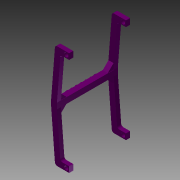
# Autodesk Inventor part: spac
Saved by Autodesk Inventor 2015 (Build 190159000, 159)
## iProperties
Created: 2015-01-15
Part Number: spac
Material: Generic
Document SubType Name: Modeling
Designer: Rafi Kurnia Putra
Density: 1 g/cm^3
Appearance: Smooth - Purple
Author: Rafi Kurnia Putra
Autodesk Inventor part; units mm, degrees
ref_plane "XZ Plane" through (0, 0, 0) normal (0, 1, 0) x (-1, 0, 0)
sketch "Sketch1" plane through (0, 0, 0) normal (0, 1, 0) x (-1, 0, 0)
  circle A0 centre (22.875, -42.175) radius 1.75
  line L0 (20.375, -39.675) -> (20.375, -44.675)
  line L1 (20.375, -44.675) -> (25.375, -44.675)
  line L2 (25.375, -44.675) -> (22.875, -44.675)
  line L3 (30.886, 0) -> (30.886, -2.5058)
  line L4 (35.886, -2.5058) -> (35.886, 0)
  line L5 (35.886, -0.0058) -> (35.886, -2.5058)
  line L6 (34.4637, -0.0058) -> (34.465, 0)
  line L7 (35.886, 0) -> (55.7448, 0) construction
  line L8 (34.4637, 0.0058) -> (34.465, 0)
  line L9 (28.0239, -37.8365) -> (30.886, -2.5058)
  line L10 (35.886, -2.5058) -> (32.6189, -42.8365)
  line L11 (25.375, -44.675) -> (30.6254, -44.675)
  line L12 (20.375, -39.675) -> (26.0305, -39.675)
  line L13 (34.4637, 0.0058) -> (34.465, 0)
  line L14 (34.4637, -0.0058) -> (34.465, 0)
  arc A1 (30.6254, -44.675) -> (32.6189, -42.8365) centre (30.6254, -42.675) ccw
  arc A2 (26.0305, -39.675) -> (28.0239, -37.8365) centre (26.0305, -37.675) ccw
  circle A3 centre (22.875, 42.175) radius 1.75
  line L15 (20.375, 39.675) -> (20.375, 44.675)
  line L16 (20.375, 44.675) -> (25.375, 44.675)
  line L17 (25.375, 44.675) -> (22.875, 44.675)
  line L18 (30.886, 0) -> (30.886, 2.5058)
  line L19 (35.886, 2.5058) -> (35.886, 0)
  line L20 (35.886, 0.0058) -> (35.886, 2.5058)
  line L21 (34.4637, 0.0058) -> (34.465, 0)
  line L22 (34.4637, -0.0058) -> (34.465, 0)
  line L23 (28.0239, 37.8365) -> (30.886, 2.5058)
  line L24 (35.886, 2.5058) -> (32.6189, 42.8365)
  line L25 (25.375, 44.675) -> (30.6254, 44.675)
  line L26 (20.375, 39.675) -> (26.0305, 39.675)
  line L27 (34.4637, -0.0058) -> (34.465, 0)
  line L28 (34.4637, 0.0058) -> (34.465, 0)
  arc A4 (32.6189, 42.8365) -> (30.6254, 44.675) centre (30.6254, 42.675) ccw
  arc A5 (28.0239, 37.8365) -> (26.0305, 39.675) centre (26.0305, 37.675) ccw
  point P0 (0, 0)
  point P1 (27.875, -39.675)
  point P2 (30.886, -2.5058)
  point P3 (35.886, -1.2558)
  point P4 (30.886, -1.2529)
  point P5 (27.875, 39.675)
  point P6 (30.886, 2.5058)
  point P7 (35.886, 1.2558)
  point P8 (30.886, 1.2529)
  dimension "d4" = 3.5
  dimension "d8" = 5
  dimension "d9" = 5
  dimension "d62" = 7.5
  dimension "d63" = 2.5
  dimension "d64" = 2
  constraints: 58 end point, 25 symmetric about line, 8 point on circle, 6 centre point, 6 coincident, 6 point on line, 4 tangent, 2 horizontal, 2 midpoint, 2 parallel, 1 equal radius, 8 other
  measures "d4" diameter of A0
  measures "d8" distance of L1.end L0.end
  measures "d9" distance of L0.start L0.end
  measures "d62" distance of L0.start point (27.875, -39.675)
  measures "d63" distance from line of L0 A0.centre
  measures "d64" radius of A1
extrude "Extrusion11" add sketch "Sketch1" along normal blind 3.5
sketch "Sketch5" plane through (0, 3.5, 0) normal (0, 1, 0) x (1, 0, 0)
  line L0 (-35.886, 2.5058) -> (-30.886, 2.5058)
  line L1 (-30.886, 2.5058) -> (-30.886, -2.4942)
  line L2 (-30.886, -2.4942) -> (-35.886, -2.4942)
  line L3 (-35.886, -2.4942) -> (-35.886, 2.5058)
  point P0 (0, 0)
  dimension "d67" = 5
  dimension "d68" = 5
  constraints: 8 end point, 2 parallel, 1 horizontal, 1 perpendicular
  measures "d67" distance of L1.end L2.end
  measures "d68" distance of L0.end L1.end
extrude "Extrusion12" add sketch "Sketch5" along normal blind 22.75
ref_plane "Work Plane10" through (-33.25, 0, 0) normal (1, 0, 0) x (0, 1, 0)
sketch "Sketch6" plane through (-33.25, 0, 0) normal (1, 0, 0) x (0, 1, 0)
  line L0 (3.5, -2.5058) -> (3.5, -7.5058)
  line L1 (3.5, -2.5058) -> (3.5, -37.8365) projected
  line L2 (3.5, -2.5058) -> (8.5, -2.5058) construction
  line L3 (3.5, -7.5058) -> (8.5, -2.5058)
  line L4 (3.5, -2.5058) -> (26.25, -2.5058) projected
  line L5 (8.5, -2.5058) -> (3.5, -2.5058)
  point P0 (0, 0)
  dimension "d72" = 5
  dimension "d73" = 90
  dimension "d74" = 45
  constraints: 8 end point, 2 perpendicular, 1 collinear, 1 horizontal, 1 point on line
  measures "d72" distance of L0.start L0.end
  measures "d73" angle of L0 L2
  measures "d74" angle of L3 L0
extrude "Extrusion13" add sketch "Sketch6" along normal mid plane 4.35
ref_plane "Work Plane11" through (0, 0, 0) normal (0, 0, 1) x (1, 0, 0)
mirror "Mirror5" about plane through (0, 0, 0) normal (0, 0, 1) of "Extrusion13"
fillet "Fillet15" radius 0.5 2 edges at (-35.886, 14.875, -2.5058) (-35.886, 14.875, 2.4942)
mirror "Mirror6" about plane through (-33.386, 26.25, -0.0058) normal (0, 1, 0) of "Extrusion11", "Extrusion12", "Extrusion13", "Mirror5", "Fillet15"
sketch "Sketch7" plane through (-35.886, 0, -2.5058) normal (-1, 0, 0) x (0, 0, 1)
  line L0 (5, 3.5) -> (5, 49) projected
  line L1 (0.5, 3.5) -> (0.5, 49) projected
  line L2 (5.0117, 52.5) -> (0, 52.5) projected
  line L3 (5.0117, 0) -> (0, 0) projected
  line L4 (0.9808, 13.1823) -> (0.9808, 13.7432)
  spline S0 degree 2 poles (0.9808, 13.7432) (0.9808, 14.304) (1.0682, 14.7016) (1.4244, 14.9521) (1.8129, 14.9521) knots 0 0 0 1 2 3 3 3
  spline S1 degree 2 poles (1.8129, 14.9521) (2.1691, 14.9521) (2.415, 14.7752) (2.4403, 14.5154) knots 0 0 0 1 2 2 2
  spline S2 degree 2 poles (2.4403, 14.5154) (2.4978, 14.7499) (2.6932, 14.9131) (2.8563, 14.9521) (3.2264, 14.9521) knots 0 0 0 1 2 3 3 3
  line L5 (3.2264, 14.9521) -> (4.0308, 14.9521)
  line L6 (4.0308, 14.9521) -> (4.0308, 14.2143)
  line L7 (4.0308, 14.2143) -> (3.0172, 14.2143)
  spline S3 degree 2 poles (3.0172, 14.2143) (2.7736, 14.2143) (2.6564, 14.1385) (2.6564, 13.9753) knots 0 0 0 1 2 2 2
  line L8 (2.6564, 13.9753) -> (4.0308, 13.9753)
  line L9 (4.0308, 13.9753) -> (4.0308, 13.1823)
  line L10 (4.0308, 13.1823) -> (0.9808, 13.1823)
  line L11 (1.5026, 13.9753) -> (2.1806, 13.9753)
  spline S4 degree 2 poles (2.1806, 13.9753) (2.1806, 14.1086) (2.1071, 14.2143) (1.9048, 14.2143) knots 0 0 0 1 2 2 2
  line L12 (1.9048, 14.2143) -> (1.737, 14.2143)
  spline S5 degree 2 poles (1.737, 14.2143) (1.5922, 14.2143) (1.5026, 14.1109) (1.5026, 13.9753) knots 0 0 0 1 2 2 2
  spline S6 degree 2 poles (2.7667, 19.1123) (3.2264, 19.1123) (3.6079, 19.0686) (3.9251, 18.8411) (4.0952, 18.4526) (4.0952, 18.1952) knots 0 0 0 1 2 3 4 4 4
  spline S7 degree 2 poles (4.0952, 18.1952) (4.0952, 17.9493) (3.9343, 17.5608) (3.6148, 17.3241) (3.2379, 17.2781) (2.7667, 17.2781) knots 0 0 0 1 2 3 4 4 4
  line L13 (2.7667, 17.2781) -> (2.245, 17.2781)
  spline S8 degree 2 poles (2.245, 17.2781) (1.7853, 17.2781) (1.4037, 17.3218) (1.0866, 17.5493) (0.9165, 17.9378) (0.9165, 18.1952) knots 0 0 0 1 2 3 4 4 4
  spline S9 degree 2 poles (0.9165, 18.1952) (0.9165, 18.4411) (1.0774, 18.8296) (1.3968, 19.0663) (1.7738, 19.1123) (2.245, 19.1123) knots 0 0 0 1 2 3 4 4 4
  line L14 (2.245, 19.1123) -> (2.7667, 19.1123)
  spline S10 degree 2 poles (1.7646, 18.3193) (1.5531, 18.3193) (1.4336, 18.2733) (1.4336, 18.1998) knots 0 0 0 1 2 2 2
  spline S11 degree 2 poles (1.4336, 18.1998) (1.4336, 18.1377) (1.5302, 18.0711) (1.7646, 18.0711) knots 0 0 0 1 2 2 2
  line L15 (1.7646, 18.0711) -> (3.1873, 18.0711)
  spline S12 degree 2 poles (3.1873, 18.0711) (3.4539, 18.0711) (3.578, 18.1148) (3.578, 18.1929) knots 0 0 0 1 2 2 2
  spline S13 degree 2 poles (3.578, 18.1929) (3.578, 18.2733) (3.4355, 18.3193) (3.1666, 18.3193) knots 0 0 0 1 2 2 2
  line L16 (3.1666, 18.3193) -> (1.7646, 18.3193)
  line L17 (0.9808, 21.4498) -> (0.9808, 22.2404)
  spline S14 degree 2 poles (0.9808, 22.2404) (0.9808, 22.6174) (1.0981, 23.0035) (1.4543, 23.2402) (1.8496, 23.2402) knots 0 0 0 1 2 3 3 3
  spline S15 degree 2 poles (1.8496, 23.2402) (2.1163, 23.2402) (2.3277, 23.0724) (2.3829, 22.8242) knots 0 0 0 1 2 2 2
  spline S16 degree 2 poles (2.3829, 22.8242) (2.4472, 23.1) (2.7345, 23.2954) (3.0333, 23.2954) knots 0 0 0 1 2 2 2
  line L18 (3.0333, 23.2954) -> (3.3137, 23.2954)
  spline S17 degree 2 poles (3.3137, 23.2954) (3.624, 23.2954) (3.9205, 23.1552) (4.0308, 22.8449) (4.0308, 22.3668) knots 0 0 0 1 2 3 3 3
  line L19 (4.0308, 22.3668) -> (4.0308, 21.4498)
  line L20 (4.0308, 21.4498) -> (0.9808, 21.4498)
  line L21 (2.6564, 22.2427) -> (3.5091, 22.2427)
  spline S18 degree 2 poles (3.5091, 22.2427) (3.5045, 22.4105) (3.4103, 22.5024) (3.2241, 22.5024) knots 0 0 0 1 2 2 2
  line L22 (3.2241, 22.5024) -> (2.9414, 22.5024)
  spline S19 degree 2 poles (2.9414, 22.5024) (2.7437, 22.5024) (2.661, 22.4197) (2.6564, 22.2427) knots 0 0 0 1 2 2 2
  line L23 (1.5026, 22.2427) -> (2.1806, 22.2427)
  spline S20 degree 2 poles (2.1806, 22.2427) (2.1783, 22.2933) (2.1783, 22.3209) knots 0 0 0 1 1 1
  spline S21 degree 2 poles (2.1783, 22.3209) (2.1783, 22.4381) (2.0634, 22.5024) (1.7922, 22.5024) knots 0 0 0 1 2 2 2
  spline S22 degree 2 poles (1.7922, 22.5024) (1.6497, 22.5024) (1.5348, 22.4496) (1.5049, 22.3645) (1.5026, 22.2427) knots 0 0 0 1 2 3 3 3
  line L24 (0.9808, 27.4233) -> (3.0195, 27.4233)
  spline S23 degree 2 poles (3.0195, 27.4233) (3.3666, 27.4233) (3.647, 27.3774) (3.9435, 27.1567) (4.0952, 26.7936) (4.0952, 26.5453) knots 0 0 0 1 2 3 4 4 4
  spline S24 degree 2 poles (4.0952, 26.5453) (4.0952, 26.2718) (3.9136, 25.8558) (3.624, 25.6467) (3.3022, 25.6099) (2.7851, 25.6099) knots 0 0 0 1 2 3 4 4 4
  line L25 (2.7851, 25.6099) -> (0.9808, 25.6099)
  line L26 (0.9808, 25.6099) -> (0.9808, 26.4028)
  line L27 (0.9808, 26.4028) -> (3.2678, 26.4028)
  spline S25 degree 2 poles (3.2678, 26.4028) (3.4677, 26.4028) (3.578, 26.4465) (3.578, 26.5109) knots 0 0 0 1 2 2 2
  spline S26 degree 2 poles (3.578, 26.5109) (3.578, 26.5867) (3.4562, 26.6304) (3.2287, 26.6304) knots 0 0 0 1 2 2 2
  line L28 (3.2287, 26.6304) -> (0.9808, 26.6304)
  line L29 (0.9808, 26.6304) -> (0.9808, 27.4233)
  line L30 (1.9025, 31.4525) -> (1.9025, 30.7147)
  line L31 (1.9025, 30.7147) -> (1.6773, 30.7147)
  spline S27 degree 2 poles (1.6773, 30.7147) (1.521, 30.7147) (1.4336, 30.6595) (1.4336, 30.5929) knots 0 0 0 1 2 2 2
  spline S28 degree 2 poles (1.4336, 30.5929) (1.4336, 30.5216) (1.5508, 30.4481) (1.6681, 30.4481) knots 0 0 0 1 2 2 2
  spline S29 degree 2 poles (1.6681, 30.4481) (1.8198, 30.4481) (1.8979, 30.4894) knots 0 0 0 1 1 1
  spline S30 degree 2 poles (1.8979, 30.4894) (1.976, 30.5308) (2.0841, 30.7147) knots 0 0 0 1 1 1
  spline S31 degree 2 poles (2.0841, 30.7147) (2.399, 31.2433) (2.6012, 31.3812) knots 0 0 0 1 1 1
  spline S32 degree 2 poles (2.6012, 31.3812) (2.8035, 31.5191) (3.2517, 31.5191) knots 0 0 0 1 1 1
  spline S33 degree 2 poles (3.2517, 31.5191) (3.578, 31.5191) (3.886, 31.3674) (4.0952, 30.9284) (4.0952, 30.6388) knots 0 0 0 1 2 3 3 3
  spline S34 degree 2 poles (4.0952, 30.6388) (4.0952, 30.3216) (3.8539, 29.8712) (3.4815, 29.731) (3.139, 29.731) knots 0 0 0 1 2 3 3 3
  line L32 (3.139, 29.731) -> (2.9391, 29.731)
  line L33 (2.9391, 29.731) -> (2.9391, 30.4687)
  line L34 (2.9391, 30.4687) -> (3.3091, 30.4687)
  spline S35 degree 2 poles (3.3091, 30.4687) (3.4792, 30.4687) (3.578, 30.5308) (3.578, 30.6089) knots 0 0 0 1 2 2 2
  spline S36 degree 2 poles (3.578, 30.6089) (3.578, 30.6894) (3.4539, 30.7652) (3.3321, 30.7652) knots 0 0 0 1 2 2 2
  spline S37 degree 2 poles (3.3321, 30.7652) (3.0632, 30.7652) (2.9805, 30.6917) knots 0 0 0 1 1 1
  spline S38 degree 2 poles (2.9805, 30.6917) (2.8977, 30.6158) (2.7023, 30.3193) knots 0 0 0 1 1 1
  spline S39 degree 2 poles (2.7023, 30.3193) (2.507, 30.0252) (2.33, 29.8321) (2.0174, 29.7057) (1.7738, 29.7057) knots 0 0 0 1 2 3 3 3
  spline S40 degree 2 poles (1.7738, 29.7057) (1.4221, 29.7057) (1.0981, 29.8849) (0.9165, 30.2849) (0.9165, 30.5676) knots 0 0 0 1 2 3 3 3
  spline S41 degree 2 poles (0.9165, 30.5676) (0.9165, 30.8756) (1.1164, 31.3123) (1.4198, 31.4525) (1.783, 31.4525) knots 0 0 0 1 2 3 3 3
  line L35 (1.783, 31.4525) -> (1.9025, 31.4525)
  line L36 (0.9808, 35.4057) -> (1.5922, 35.4057)
  line L37 (1.5922, 35.4057) -> (1.5922, 34.9346)
  line L38 (1.5922, 34.9346) -> (4.0308, 34.9346)
  line L39 (4.0308, 34.9346) -> (4.0308, 34.1416)
  line L40 (4.0308, 34.1416) -> (1.5922, 34.1416)
  line L41 (1.5922, 34.1416) -> (1.5922, 33.6727)
  line L42 (1.5922, 33.6727) -> (0.9808, 33.6727)
  line L43 (0.9808, 33.6727) -> (0.9808, 35.4057)
  line L44 (0.9808, 38.9982) -> (4.0308, 39.4533)
  line L45 (4.0308, 39.4533) -> (4.0308, 38.6396)
  line L46 (4.0308, 38.6396) -> (3.4815, 38.5982)
  line L47 (3.4815, 38.5982) -> (3.4815, 38.3155)
  line L48 (3.4815, 38.3155) -> (4.0308, 38.2696)
  line L49 (4.0308, 38.2696) -> (4.0308, 37.4467)
  line L50 (4.0308, 37.4467) -> (0.9808, 37.849)
  line L51 (0.9808, 37.849) -> (0.9808, 38.9982)
  spline S42 degree 2 poles (2.9414, 38.5776) (2.4242, 38.5201) (1.6612, 38.458) knots 0 0 0 1 1 1
  spline S43 degree 2 poles (1.6612, 38.458) (2.5369, 38.3385) (2.9414, 38.3063) knots 0 0 0 1 1 1
  line L52 (2.9414, 38.3063) -> (2.9414, 38.5776)
  point P0 (2.5058, 0)
  point P1 (2.5058, 26.25)
  point P2 (5, 26.25)
  point P3 (2.5058, 26.25)
  point P4 (2.5058, 26.25)
  dimension "d81" = 22.75
  constraints: 2 coincident, 1 midpoint, 2 other
  measures "d81" distance of L0.end point (5, 26.25)
extrude "Extrusion14" add sketch "Sketch7" along normal blind 1
body "Solid4"
